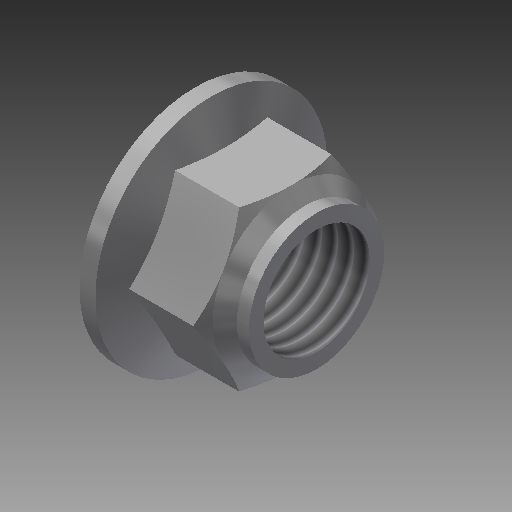
# Autodesk Inventor part: 314-11
Saved by Autodesk Inventor 2019 (Build 230136000, 136)
## iProperties
Company: Autodesk Inc.
Created: 2007-10-30
Part Number: 314-11
Document SubType Name: Modeling
Designer: Autodesk Inc.
Density: 7.85 g/cm^3
Mass: 12.3234 g
Surface Area: 14.5331 cm^2
Volume: 1.56986 cm^3
Material: Steel, Mild
Description: NUT R2456 - M12
Appearance: Steel
Component Category: Fasteners
Author: Inventor
Autodesk Inventor part; units mm, degrees
ref_plane "YZ Plane" through (0, 0, 0) normal (1, 0, 0) x (0, 1, 0)
ref_plane "XZ Plane" through (0, 0, 0) normal (0, 1, 0) x (-1, 0, 0)
ref_plane "XY Plane" through (0, 0, 0) normal (0, 0, 1) x (1, 0, 0)
sketch "Sketch2" plane through (0, 0, 0) normal (1, 0, 0) x (0, 1, 0)
  line L0 (-7.5, 4.3301) -> (0, 8.6603)
  line L1 (0, 8.6603) -> (7.5, 4.3301)
  line L2 (7.5, 4.3301) -> (7.5, -4.3301)
  line L3 (7.5, -4.3301) -> (0, -8.6603)
  line L4 (0, -8.6603) -> (-7.5, -4.3301)
  line L5 (-7.5, -4.3301) -> (-7.5, 4.3301)
  line L6 (0, 12.1244) -> (0, -12.1244) projected
  circle A0 centre (0, 0) radius 5
  dimension "d1" = 10
  constraints: 12 end point, 2 coincident, 1 centre point, 1 parallel, 13 other
  measures "d1" diameter of A0
extrude "Extrusion1" add sketch "Sketch2" along normal blind 11.4 contours L0 L6 A0 L4 L5 | L1 L2 L3 L6 A0
sketch "Sketch3" plane through (0, 0, 0) normal (0, 0, 1) x (1, 0, 0)
  line L0 (0, 10.9) -> (0, -10.9) projected
  line L1 (0, -10.9) -> (0, -5)
  line L2 (0, -10.9) -> (1.5, -10.9)
  line L3 (1.5, -10.9) -> (3.9439, -5)
  line L4 (3.9439, -5) -> (0, -5)
  line L5 (-0.7888, 0) -> (4.7326, 0) projected
  point P0 (0, 0)
  dimension "d4" = 1.5
  dimension "d5" = 22.5
  dimension "d6" = 5
  constraints: 8 end point, 2 perpendicular, 1 point on line
  measures "d4" distance of L0.end L2.end
  measures "d5" angle of L0 L3
  measures "d6" distance from line of point (0, 0) L4
revolve "Revolution1" add sketch "Sketch3" angle 360 about axis through (0, 0, 0) along (1, 0, 0)
sketch "Sketch4" plane through (0, 0, 0) normal (0, 1, 0) x (-1, 0, 0)
  line L0 (-11.4, 4.3301) -> (-11.4, 8.6603) projected
  line L1 (-11.4, 6.36) -> (-10.26, 6.36)
  line L2 (-10.26, 6.36) -> (-9.12, 7.5)
  line L3 (-9.12, 7.5) -> (-8.0461, 9.36)
  line L4 (-8.0461, 9.36) -> (-11.4, 9.36)
  line L5 (-11.4, 9.36) -> (-11.4, 6.36)
  line L6 (-9.12, 7.5) -> (-10.26, 6.36)
  line L7 (-8.4501, 8.6603) -> (-9.12, 7.5)
  line L8 (2.28, 0) -> (-13.68, 0) projected
  point P0 (0, 0)
  dimension "d8" = 135
  dimension "d9" = 1.14
  dimension "d10" = 6.36
  dimension "d11" = 120
  dimension "d12" = 2.28
  dimension "d13" = 3
  constraints: 14 end point, 2 perpendicular, 1 parallel, 1 point on line, 6 other
  measures "d8" angle of L1 L2
  measures "d9" distance of L1.start L1.end
  measures "d10" distance from line of point (0, 0) L1
  measures "d11" angle of L1 L3
  measures "d12" distance from line of L2.end L0
  measures "d13" distance of L4.end L1.start
revolve "Revolution2" cut sketch "Sketch4" angle 360 about axis through (-10, 0, 0) along (1, 0, 0)
thread "Thread1" size "M10x1.5" class "6H" standard "ANSI Metric M Profile" full length
body "Solid1"
